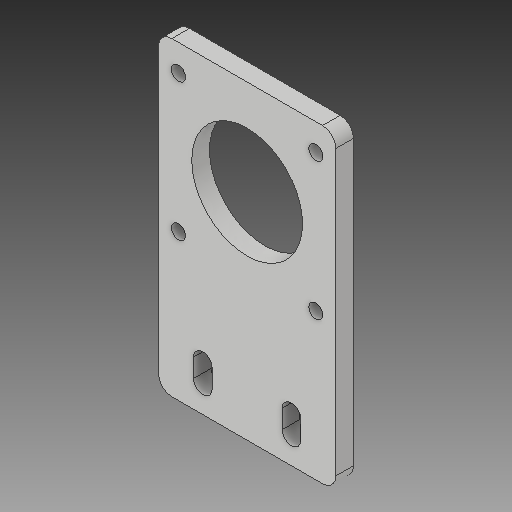
# Autodesk Inventor part: nema17-mount-bottom-z-axis-v2
Saved by Autodesk Inventor 2018 (Build 220112000, 112)
## iProperties
Created: 2017-11-04
Part Number: nema17-mount-bottom-z-axis-v2
Material: Generic
Document SubType Name: Modeling
Designer: Jurjen
Density: 1 g/cm^3
Appearance: Default
Author: Jurjen
Autodesk Inventor part; units mm, degrees
ref_plane "YZ Plane" through (0, 0, 0) normal (1, 0, 0) x (0, 1, 0)
ref_plane "XZ Plane" through (0, 0, 0) normal (0, 1, 0) x (-1, 0, 0)
ref_plane "XY Plane" through (0, 0, 0) normal (0, 0, 1) x (1, 0, 0)
sketch "Sketch1" plane through (0, 0, 0) normal (0, 0, 1) x (1, 0, 0)
  line L0 (-20, 35) -> (20, 35)
  line L1 (20, 35) -> (20, -35)
  line L2 (20, -35) -> (-20, -35)
  line L3 (-20, -35) -> (-20, 35)
  point P0 (0, 0)
  point P1 (0, 35)
  point P2 (20, 0)
  dimension "d0" = 40
  dimension "d1" = 70
  constraints: 8 end point, 2 midpoint, 2 parallel, 1 horizontal, 1 horizontal alignment, 1 perpendicular, 1 vertical alignment
  measures "d0" distance between parallel lines of L3 L1
  measures "d1" distance between parallel lines of L2 L0
extrude "Extrusion1" add sketch "Sketch1" along normal mid plane 4
sketch "Sketch2" plane through (0, 0, 2) normal (0, 0, 1) x (1, 0, 0)
  circle A0 centre (0, 13.5) radius 12.5
  circle A1 centre (-15.5, 29) radius 1.6
  circle A2 centre (15.5, 29) radius 1.6
  circle A3 centre (15.5, -2) radius 1.6
  circle A4 centre (-15.5, -2) radius 1.6
  line L0 (-15.5, 29) -> (15.5, 29) construction
  line L1 (20, 35) -> (-20, 35) projected
  line L2 (-15.5, -2) -> (-15.5, 29) construction
  point P0 (0, 0)
  point P1 (0, 29)
  point P2 (-15.5, 13.5)
  dimension "d4" = 3.2
  dimension "d5" = 31
  dimension "d6" = 31
  dimension "d7" = 21.5
  dimension "d8" = 25
  constraints: 5 centre point, 4 end point, 4 vertical alignment, 3 equal radius, 3 horizontal alignment, 2 midpoint, 1 horizontal, 1 vertical
  measures "d4" diameter of A1
  measures "d5" distance of L0.end L0.start
  measures "d6" distance of L0.start L2.start
  measures "d7" distance from line of L1 A0.centre
  measures "d8" diameter of A0
extrude "Extrusion2" cut sketch "Sketch2" against normal up to next
sketch "Sketch3" plane through (0, 0, 2) normal (0, 0, 1) x (1, 0, 0)
  arc A0 (-7.9, -24.8) -> (-12.1, -24.8) centre (-10, -24.8) ccw
  arc A1 (12.1, -24.8) -> (7.9, -24.8) centre (10, -24.8) ccw
  line L0 (-10, -24.8) -> (10, -24.8) construction
  arc A2 (-12.1, -29) -> (-7.9, -29) centre (-10, -29) ccw
  arc A3 (7.9, -29) -> (12.1, -29) centre (10, -29) ccw
  line L1 (-12.1, -29) -> (-12.1, -24.8)
  line L2 (-7.9, -24.8) -> (-7.9, -29)
  line L3 (7.9, -24.8) -> (7.9, -29)
  line L4 (12.1, -29) -> (12.1, -24.8)
  line L5 (-20, -35) -> (20, -35) projected
  point P0 (0, 0)
  point P1 (0, -24.8)
  dimension "d11" = 4.2
  dimension "d12" = 4.2
  dimension "d13" = 20
  dimension "d14" = 6
  constraints: 10 end point, 8 point on circle, 6 tangent, 4 centre point, 3 equal radius, 3 parallel, 2 point on line, 1 horizontal, 1 horizontal alignment, 1 midpoint, 1 vertical, 1 vertical alignment
  measures "d11" diameter of A0
  measures "d12" distance of L0.start A2.centre
  measures "d13" distance of L0.end L0.start
  measures "d14" distance from line of L5 A2.centre
extrude "Extrusion3" cut sketch "Sketch3" against normal up to next
fillet "Fillet1" radius 3 4 edges at (-20, -35, 0) (20, -35, 0) (20, 35, 0) (-20, 35, 0)
equation "\"d6\" = d5"
body "Solid1"
